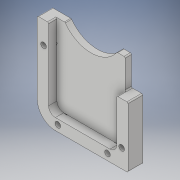
# Autodesk Inventor part: high_leg_teflon
Saved by Autodesk Inventor 2018 (Build 220112000, 112)
## iProperties
Created: 2018-03-29
Part Number: high_leg_teflon
Material: Generic
Document SubType Name: Modeling
Designer: etd
Density: 1 g/cm^3
Appearance: Default
Vendor: Rhoban
Mass: 5.58553 g
Surface Area: 43.312 cm^2
Volume: 5.58553 cm^3
Author: etd
Autodesk Inventor part; units mm, degrees
ref_plane "YZ Plane" through (0, 0, 0) normal (1, 0, 0) x (0, 1, 0)
ref_plane "XZ Plane" through (0, 0, 0) normal (0, 1, 0) x (-1, 0, 0)
ref_plane "XY Plane" through (0, 0, 0) normal (0, 0, 1) x (1, 0, 0)
sketch "Sketch2" plane through (0, 0, 0) normal (0, 0, 1) x (1, 0, 0)
  line L0 (0, 0) -> (5, 0) construction
  line L1 (40.2, 0) -> (40.2, -40)
  line L2 (40.2, -40) -> (0, -40)
  line L3 (0, -40) -> (0, -13.1)
  arc A0 (31.6412, 0) -> (8.5588, 0) centre (20.1, 8.1) ccw construction
  line L4 (31.6412, 0) -> (40.2, 0)
  line L5 (8.5588, 0) -> (31.6412, 0) construction
  arc A1 (8.5588, 0) -> (31.6412, 0) centre (20.1, 8.1) ccw
  line L6 (35.2, 0) -> (31.6412, 0)
  line L7 (5, 0) -> (5, -13.1)
  line L8 (5, -35) -> (35.2, -35)
  line L9 (35.2, -35) -> (35.2, 0)
  line L10 (0, -13.1) -> (5, -13.1)
  line L11 (0, -13.1) -> (0, 0) construction
  line L12 (5, -13.1) -> (5, -35)
  line L13 (5, 0) -> (8.5588, 0)
  line L14 (8.5588, 0) -> (5, 0)
  line L15 (31.6412, 0) -> (8.5588, 0) construction
  line L16 (20.1, 0) -> (20.1, 8.1)
  line L17 (31.1, -37.2) -> (40.2, -37.2) construction
  line L18 (9.1, -37.2) -> (0, -37.2) construction
  point P0 (2.8, -31.9)
  point P1 (37.4, -9.9)
  dimension "d0" = 40
  dimension "d1" = 40.2
  dimension "d55" = 28.2
  dimension "d56" = 5
  dimension "d57" = 5
  dimension "d58" = 5
  dimension "d59" = 26.9
  dimension "d66" = 48.1
  dimension "d67" = 2.8
  dimension "d68" = 2.8
  dimension "d69" = 2.8
  dimension "d70" = 22
  dimension "d72" = 30.1
  dimension "d73" = 8.1
  dimension "d74" = 2.8
  constraints: 38 end point, 14 perpendicular, 11 parallel, 7 horizontal, 4 point on circle, 3 point on line, 2 centre point, 2 collinear, 1 coincident, 1 midpoint, 1 vertical
  measures "d0" distance of L1.start L1.end
  measures "d1" distance of L0.start L1.start
  measures "d55" diameter of A0
  measures "d56" distance between parallel lines of L1 L9
  measures "d57" distance between parallel lines of L3 L7
  measures "d58" distance between parallel lines of L8 L2
  measures "d59" distance from line of L3.end L2
  measures "d66" distance from line of L16.end L2
  measures "d67" distance from line of L2 L17.start
  measures "d68" distance from line of L2 L18.start
  measures "d69" distance from line of L1 point (37.4, -9.9)
  measures "d70" distance of L18.start L17.start
  measures "d72" distance from line of point (37.4, -9.9) L2
  measures "d73" distance from line of L2 point (2.8, -31.9)
  measures "d74" distance from line of L3 point (2.8, -31.9)
extrude "Extrusion6" add sketch "Sketch2" along normal blind 6.5 contours L1 L2 L3 L10 L12 L8 L9 L4
extrude "Extrusion8" add sketch "Sketch2" along normal blind 2.8 contours L9 L8 L12 L7 L13 A1 L4
hole "Hole2" at (20.1, 8.1, 0) at (31.1, -37.2, 0) at (9.1, -37.2, 0) at (2.8, -31.9, 0) at (37.4, -9.9, 0) direction (0, 0, 1) diameter 2.5 end through all counterbore diameter 4.5 counterbore depth 3
fillet "Fillet1" radius 0.5 9 edges at (40.2, 0, 3.25) (35.2, 0, 4.65) (5, -13.1, 4.65) (5, -13.1, 1.4) (0, -13.1, 3.25) (0, -40, 3.25) (31.6412, 0, 1.4) (8.5588, 0, 1.4) (5, 0, 1.4)
fillet "Fillet2" radius 3 2 edges at (35.2, -35, 4.65) (5, -35, 4.65)
fillet "Fillet3" radius 8 1 edges at (40.2, -40, 3.25)
mirror "Mirror2" about plane through (40.2, -40, 0) normal (1, 0, 0) remove original yes
equation "\"d1\" = side_to_side_outside_dist"
equation "\"d56\" = outside_inside_dist - tol"
equation "\"d57\" = outside_inside_dist - tol"
equation "\"d58\" = outside_inside_dist - tol"
equation "\"d66\" = front_to_axe"
equation "\"d67\" = holes_to_side"
equation "\"d68\" = holes_to_side"
equation "\"d69\" = holes_to_side"
equation "\"d74\" = holes_to_side"
equation "\"d60\" = outside_depth"
equation "\"outside_inside_dist\" = 5.1"
equation "\"outside_depth\" = 6.5"
equation "\"inside_depth\" = outside_depth - outside_to_inside"
equation "\"tol\" = 0.1"
equation "\"side_to_side_outside_dist\" = 40.2"
equation "\"front_to_torsebas\" = 27.1"
equation "\"front_to_axe\" = 48.1"
equation "\"palonnier_diameter\" = 28"
equation "\"holes_to_side\" = 2.8"
equation "\"outside_to_inside\" = 3.5"
body "Solid2"
